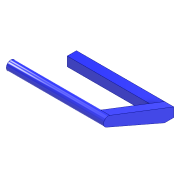
# Autodesk Inventor part: Radius_Bone1_Joint
Saved by Autodesk Inventor 2020 (Build 240168000, 168)
## iProperties
Created: 2021-03-04
Part Number: Radius_Bone1_Joint
Material: Generic
Document SubType Name: Modeling
Designer: deox
Density: 1 g/cm^3
Appearance: Blue - Wall Paint - Glossy
Author: deox
Autodesk Inventor part; units mm, degrees
ref_plane "YZ Plane" through (0, 0, 0) normal (1, 0, 0) x (0, 1, 0)
ref_plane "XZ Plane" through (0, 0, 0) normal (0, 1, 0) x (-1, 0, 0)
ref_plane "XY Plane" through (0, 0, 0) normal (0, 0, 1) x (1, 0, 0)
sketch "Sketch1" plane through (0, 0, 0) normal (1, 0, 0) x (0, 1, 0)
  line L0 (0, 0) -> (2.696, 0)
  line L1 (2.696, 0) -> (2.696, 6.6)
  circle A0 centre (2.696, 6.6) radius 0.5
  line L2 (-0.5, 0.5) -> (0.5, 0.5)
  line L3 (0.5, 0.5) -> (0.5, -0.5)
  line L4 (0.5, -0.5) -> (-0.5, -0.5)
  line L5 (-0.5, -0.5) -> (-0.5, 0.5)
  line L6 (-0.5, 0.5) -> (0.5, -0.5) construction
  line L7 (0.5, 0.5) -> (-0.5, -0.5) construction
  line L8 (0.5, -0.5) -> (3.1627, 6.4205)
  line L9 (-0.5, 0.5) -> (2.2374, 6.7993)
  dimension "d0" = 2.696
  dimension "d1" = 6.6
  dimension "d2" = 1
  dimension "d3" = 1
  dimension "d4" = 1
  constraints: 20 end point, 2 horizontal, 2 midpoint, 2 parallel, 2 perpendicular, 2 point on circle, 2 tangent, 1 centre point, 1 coincident
  measures "d0" distance of L0.start L0.end
  measures "d1" distance of L0.end L1.end
  measures "d2" diameter of A0
  measures "d3" distance of L3.end L4.end
  measures "d4" distance of L2.end L3.end
extrude "Extrusion1" add sketch "Sketch1" along normal blind 1 contours L3 L2 L9 A0 L1 L8 L0 | L3 L4 L5 L2 | L0 L8 L3 | L1 A0 L8 | A0
sketch "Sketch2" plane through (0, 0, 0) normal (-1, 0, 0) x (0, 0, 1)
  line L0 (-0.5, -0.5) -> (0.5, -0.5)
  line L1 (0.5, -0.5) -> (0.5, 0.5)
  line L2 (0.5, 0.5) -> (-0.5, 0.5)
  line L3 (-0.5, 0.5) -> (-0.5, -0.5)
  line L4 (-0.5, -0.5) -> (0.5, 0.5) construction
  line L5 (0.5, -0.5) -> (-0.5, 0.5) construction
  arc A0 (6.7993, 2.2374) -> (6.4205, 3.1627) centre (6.6, 2.696) ccw projected
  circle A1 centre (6.6, 2.696) radius 0.5
  point P0 (0, 0)
  point P1 (6.4205, 3.1627)
  point P2 (6.7993, 2.2374)
  dimension "d7" = 1
  dimension "d8" = 1
  constraints: 12 end point, 2 midpoint, 2 parallel, 1 centre point, 1 coincident, 1 horizontal, 1 perpendicular
  measures "d7" distance of L2.end L1.end
  measures "d8" distance of L1.end L0.end
extrude "Extrusion2" add sketch "Sketch2" along normal blind 9.53
body "Solid1"
